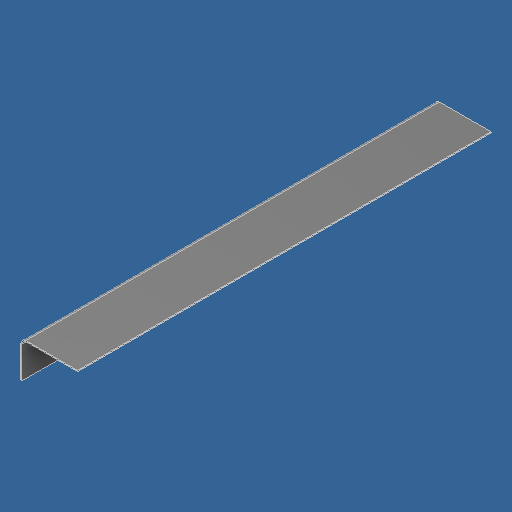
# Autodesk Inventor part: TopPlate
Saved by Autodesk Inventor 2023 (Build 270158030, 158C)
## iProperties
Created: 2022-11-17
Part Number: TopPlate
Material: ABS Plastic
Document SubType Name: Modeling
Designer: kumpu
Density: 1.06 g/cm^3
Appearance: Smooth - Black
Mass: 160.66 g
Surface Area: 1935.06 cm^2
Volume: 151.566 cm^3
Author: kumpu
Autodesk Inventor part; units mm, degrees
ref_plane "YZ Plane" through (0, 0, 0) normal (1, 0, 0) x (0, 1, 0)
ref_plane "XZ Plane" through (0, 0, 0) normal (0, 1, 0) x (-1, 0, 0)
ref_plane "XY Plane" through (0, 0, 0) normal (0, 0, 1) x (1, 0, 0)
sketch "Sketch1" plane through (0, 0, 0) normal (0, 1, 0) x (-1, 0, 0)
  line L0 (41.275, 330.2) -> (-41.275, 330.2)
  line L1 (-41.275, 330.2) -> (-41.275, -330.2)
  line L2 (-41.275, -330.2) -> (41.275, -330.2)
  line L3 (41.275, -330.2) -> (41.275, 330.2)
  line L4 (41.275, 330.2) -> (-41.275, -330.2) construction
  line L5 (-41.275, 330.2) -> (41.275, -330.2) construction
  point P0 (0, 0)
  dimension "d0" = 82.55
  dimension "d1" = 660.4
  constraints: 12 end point, 2 midpoint, 2 parallel, 1 horizontal, 1 perpendicular
  measures "d0" distance of L2.end L1.end
  measures "d1" distance of L1.end L0.end
extrude "Extrusion1" add sketch "Sketch1" along normal mid plane 1.5875
sketch "Sketch2" plane through (41.275, 0.7937, -330.2) normal (0, 0, -1) x (-1, 0, 0)
  line L0 (90.4875, -7.9375) -> (90.4875, -58.7375)
  line L1 (90.4875, -58.7375) -> (88.9, -58.7375)
  line L2 (88.9, -58.7375) -> (88.9, -7.9375)
  arc A0 (88.9, -7.9375) -> (82.55, -1.5875) centre (82.55, -7.9375) ccw
  line L3 (82.55, -1.5875) -> (82.55, 0)
  arc A1 (90.4875, -7.9375) -> (82.55, 0) centre (82.55, -7.9375) ccw
  point P0 (41.275, -0.7937)
  dimension "d4" = 6.35
  dimension "d5" = 57.15
  dimension "d6" = 1.5875
  constraints: 8 end point, 4 point on circle, 2 centre point, 2 line through centre, 2 perpendicular, 2 tangent, 1 coincident, 1 concentric, 1 parallel, 1 point on line, 1 vertical
  measures "d4" radius of A0
  measures "d5" distance from line of L1 L3.start
  measures "d6" distance of L3.start L3.end
extrude "Extrusion2" add sketch "Sketch2" against normal blind 660.4
body "Solid1"
